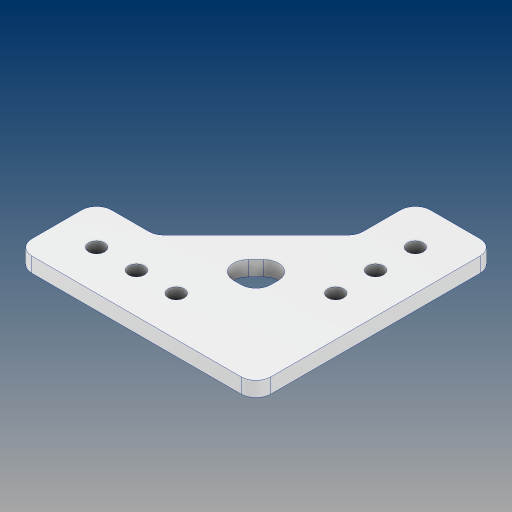
# Autodesk Inventor part: ELEV_008_SUPBRK3
Saved by Autodesk Inventor 2024.3 (Build 283343000, 343)
## iProperties
Created: 2024-11-25
Part Number: ELEV_008_SUPBRK3
Material: Aluminum 6061
Document SubType Name: Modeling
Designer: Kenji
Density: 2.7 g/cm^3
Appearance: Aluminum - Flat
Author: Kenji
Autodesk Inventor part; units mm, degrees
ref_plane "YZ Plane" through (0, 0, 0) normal (1, 0, 0) x (0, 1, 0)
ref_plane "XZ Plane" through (0, 0, 0) normal (0, 1, 0) x (-1, 0, 0)
ref_plane "XY Plane" through (0, 0, 0) normal (0, 0, 1) x (1, 0, 0)
sketch "Sketch1" plane through (0, 0, 0) normal (0, 1, 0) x (-1, 0, 0)
  line L0 (0, -4.7625) -> (0, -71.4375)
  line L1 (4.7625, -76.2) -> (20.6375, -76.2)
  line L2 (4.7625, 0) -> (71.4375, 0)
  line L3 (76.2, -4.7625) -> (76.2, -20.6375)
  circle A0 centre (12.7, -38.1) radius 2.54
  circle A1 centre (12.7, -50.8) radius 2.54
  circle A2 centre (12.7, -63.5) radius 2.54
  line L4 (12.7, -76.2) -> (12.7, 0) construction
  circle A3 centre (63.5, -12.7) radius 2.54
  circle A4 centre (50.8, -12.7) radius 2.54
  circle A5 centre (38.1, -12.7) radius 2.54
  line L5 (76.2, -12.7) -> (0, -12.7) construction
  line L6 (61.7039, -14.4961) -> (14.4961, -61.7039) construction
  line L7 (56.1403, -26.7949) -> (26.7949, -56.1403)
  line L8 (35.9347, -33.5301) -> (33.5301, -35.9347)
  line L9 (25.4, -32.5671) -> (25.4, -30.1625)
  line L10 (30.1625, -25.4) -> (32.5671, -25.4)
  line L11 (25.4, -71.4375) -> (25.4, -59.5079)
  line L12 (71.4375, -25.4) -> (59.5079, -25.4)
  arc A6 (76.2, -4.7625) -> (71.4375, 0) centre (71.4375, -4.7625) ccw
  arc A7 (71.4375, -25.4) -> (76.2, -20.6375) centre (71.4375, -20.6375) ccw
  arc A8 (59.5079, -25.4) -> (56.1403, -26.7949) centre (59.5079, -30.1625) ccw
  arc A9 (26.7949, -56.1403) -> (25.4, -59.5079) centre (30.1625, -59.5079) ccw
  arc A10 (0, -71.4375) -> (4.7625, -76.2) centre (4.7625, -71.4375) ccw
  arc A11 (20.6375, -76.2) -> (25.4, -71.4375) centre (20.6375, -71.4375) ccw
  arc A12 (35.9347, -33.5301) -> (32.5671, -25.4) centre (32.5671, -30.1625) ccw
  arc A13 (25.4, -32.5671) -> (33.5301, -35.9347) centre (30.1625, -32.5671) ccw
  arc A14 (30.1625, -25.4) -> (25.4, -30.1625) centre (30.1625, -30.1625) ccw
  arc A15 (4.7625, 0) -> (0, -4.7625) centre (4.7625, -4.7625) ccw
  point P0 (0, 0)
  point P1 (0, -76.2)
  point P2 (25.4, -76.2)
  point P3 (76.2, 0)
  point P4 (76.2, -25.4)
  dimension "d3" = 5.08
  dimension "d0" = 25.4
  dimension "d1" = 76.2
  dimension "d2" = 76.2
  dimension "d4" = 12.7
  dimension "d5" = 12.7
  dimension "d6" = 12.7
  dimension "d7" = 38.1
  dimension "d9" = 12.7
  dimension "d10" = 12.7
  dimension "d11" = 38.1
  dimension "d12" = 4.7625
  dimension "d13" = 4.7625
  dimension "d14" = 4.7625
  dimension "d15" = 4.7625
  dimension "d16" = 4.7625
  dimension "d17" = 4.7625
  constraints: 26 end point, 20 point on circle, 20 point on line, 20 tangent, 14 centre point, 8 equal radius, 5 perpendicular, 4 midpoint, 4 vertical, 2 horizontal, 2 parallel, 9 other
  measures "d0" distance of point (76.2, 0) point (76.2, -25.4)
  measures "d1" distance of point (0, 0) point (0, -76.2)
  measures "d2" distance of point (0, 0) point (76.2, 0)
  measures "d4" distance between parallel lines of L0 L4
  measures "d5" distance of A1.centre A0.centre
  measures "d6" distance of point (12.7, -63.5) A1.centre
  measures "d7" distance from line of L2 A0.centre
  measures "d9" distance of A5.centre A4.centre
  measures "d10" distance of A4.centre point (63.5, -12.7)
  measures "d11" distance from line of L0 A5.centre
  measures "d12" distance between parallel lines of L6 L7
  measures "d13" distance between parallel lines of L6 L8
  measures "d14" radius of A6
  measures "d15" radius of A10
  measures "d16" radius of A12
  measures "d17" radius of A15
extrude "Extrusion1" add sketch "Sketch1" along normal blind 4.7625
body "Solid1"
